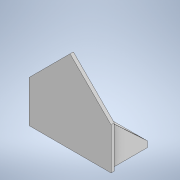
# Autodesk Inventor part: Halterung_ID6
Saved by Autodesk Inventor 2022.2 (Build 262287010, 287A)
## iProperties
Created: 2024-02-12
Part Number: Halterung_ID6
Material: Generisch
Document SubType Name: Modeling
Designer: ppovolni
Density: 1 g/cm^3
Appearance: Vorgabe
Author: ppovolni
Autodesk Inventor part; units mm, degrees
ref_plane "YZ Plane" through (0, 0, 0) normal (1, 0, 0) x (0, 1, 0)
ref_plane "XZ Plane" through (0, 0, 0) normal (0, 1, 0) x (-1, 0, 0)
ref_plane "XY Plane" through (0, 0, 0) normal (0, 0, 1) x (1, 0, 0)
sketch "Skizze1" plane through (0, 0, 0) normal (0, 0, 1) x (1, 0, 0)
  line L0 (0, 113.1371) -> (56.5685, 56.5685)
  line L1 (56.5685, 56.5685) -> (0, 0) construction
  line L2 (0, 0) -> (-56.5685, 56.5685) construction
  line L3 (-56.5685, 56.5685) -> (0, 113.1371)
  line L4 (0, 0) -> (-109.9706, 0) construction
  line L5 (-56.5685, 56.5685) -> (-56.5685, 0)
  line L6 (56.5685, 56.5685) -> (56.5685, 0)
  line L7 (-56.5685, 0) -> (56.5685, 0)
  dimension "d0" = 45
  dimension "d1" = 80
  constraints: 16 end point, 3 perpendicular, 2 horizontal, 2 parallel, 1 coincident, 1 point on line, 1 vertical
  measures "d0" angle of L4 L2
  measures "d1" distance of L0.end L1.end
extrude "Extrusion1" add sketch "Skizze1" along normal blind 5
sketch "Skizze2" plane through (0, 0, 0) normal (0, 0, -1) x (-1, 0, 0)
  line L0 (-56.5685, 0) -> (56.5685, 0)
  line L1 (56.5685, 0) -> (56.5685, 5)
  line L2 (56.5685, 5) -> (-56.5685, 5)
  line L3 (-56.5685, 5) -> (-56.5685, 0)
  line L4 (56.5685, 0) -> (-56.5685, 0) construction
  line L5 (56.5685, 56.5685) -> (56.5685, 0) construction
  line L6 (0, 113.1371) -> (56.5685, 56.5685) construction
  line L7 (-56.5685, 56.5685) -> (0, 113.1371) construction
  line L8 (-56.5685, 0) -> (-56.5685, 56.5685) construction
  point P0 (0, 0)
  dimension "d4" = 5
  constraints: 8 end point, 2 parallel, 1 collinear, 1 horizontal, 1 perpendicular
  measures "d4" distance between parallel lines of L0 L2
extrude "Extrusion2" add sketch "Skizze2" along normal blind 55
sketch "Skizze3" plane through (56.5685, 0, 5) normal (1, 0, 0) x (0, 0, -1)
  line L0 (5, 5) -> (5, 56.5685) construction
  line L1 (5, 5) -> (60, 5) construction
  line L2 (5, 56.5685) -> (60, 5)
  line L3 (60, 5) -> (5, 5)
  line L4 (5, 5) -> (5, 56.5685)
  point P0 (5, 0)
  constraints: 6 end point, 1 horizontal
extrude "Extrusion3" add sketch "Skizze3" against normal blind 5
sketch "Skizze4" plane through (-56.5685, 0, 5) normal (-1, 0, 0) x (0, 0, 1)
  line L0 (-5, 5) -> (-60, 5) projected
  line L1 (-5, 56.5685) -> (-5, 5) projected
  line L2 (-5, 56.5685) -> (-60, 5) projected
  point P0 (-5, 0)
extrude "Extrusion4" add sketch "Skizze4" against normal blind 5
sketch "Skizze5" plane through (51.5685, 5, 0) normal (0, 1, 0) x (1, 0, 0)
  line L0 (-15, 35) -> (-88.1371, 35) construction
  line L1 (-15, 38.1623) -> (-88.1371, 38.1623)
  line L2 (-88.1371, 31.8377) -> (-15, 31.8377)
  arc A0 (-15, 31.8377) -> (-15, 38.1623) centre (-15, 35) ccw
  arc A1 (-88.1371, 38.1623) -> (-88.1371, 31.8377) centre (-88.1371, 35) ccw
  line L3 (-103.1371, 55) -> (-103.1371, 0) construction
  line L4 (0, 0) -> (-103.1371, 0) construction
  line L5 (0, 0) -> (0, 55) construction
  line L6 (-103.1371, 55) -> (0, 55) construction
  point P0 (-51.5685, 0)
  point P1 (-51.5685, 35)
  dimension "d11" = 20
  dimension "d12" = 15
  dimension "d13" = 15
  constraints: 8 end point, 4 point on circle, 4 tangent, 2 centre point, 1 horizontal, 1 midpoint, 1 parallel
  measures "d11" distance between parallel lines of L6 L0
  measures "d12" distance from line of L5 L0.start
  measures "d13" distance from line of L0.end L3
extrude "Extrusion5" cut sketch "Skizze5" against normal through all
sketch "Skizze6" plane through (0, 0, 5) normal (0, 0, 1) x (1, 0, 0)
  line L0 (-56.5685, 0) -> (56.5685, 0) projected
  line L1 (56.5685, 0) -> (56.5685, 56.5685) projected
  line L2 (56.5685, 56.5685) -> (0, 113.1371) projected
  line L3 (0, 113.1371) -> (-56.5685, 56.5685) projected
  line L4 (-56.5685, 56.5685) -> (-56.5685, 0) projected
  line L5 (-61.5685, 58.6396) -> (0, 120.2082)
  line L6 (0, 120.2082) -> (61.5685, 58.6396)
  line L7 (61.5685, 58.6396) -> (61.5685, -4)
  line L8 (-61.5685, 58.6396) -> (-61.5685, -4)
  line L9 (-61.5685, -4) -> (61.5685, -4)
  line L10 (56.5685, 56.5685) -> (0, 113.1371) projected
  line L11 (-56.5685, 0) -> (56.5685, 0) projected
  point P0 (0, 0)
  dimension "d16" = 5
  dimension "d17" = 5
  dimension "d18" = 5
  dimension "d19" = 5
  dimension "d20" = 4
  constraints: 10 end point, 5 parallel, 1 perpendicular
  measures "d16" distance between parallel lines of L2 L6
  measures "d17" distance between parallel lines of L1 L7
  measures "d18" distance between parallel lines of L3 L5
  measures "d19" distance between parallel lines of L8 L4
  measures "d20" distance between parallel lines of L9 L0
extrude "Extrusion6" add sketch "Skizze6" against normal up to surface (5 mm away)
sketch "Skizze7" plane through (-56.5685, 0, 0) normal (0, -1, 0) x (1, 0, 0)
  line L0 (113.1371, 0) -> (0, 0) projected
  line L1 (0, 0) -> (0, -55) projected
  line L2 (113.1371, -55) -> (0, -55) projected
  line L3 (113.1371, -55) -> (113.1371, 0) projected
  line L4 (20, -31.8377) -> (93.1371, -31.8377) projected
  arc A0 (93.1371, -38.1623) -> (93.1371, -31.8377) centre (93.1371, -35) ccw projected
  line L5 (93.1371, -38.1623) -> (20, -38.1623) projected
  arc A1 (20, -31.8377) -> (20, -38.1623) centre (20, -35) ccw projected
  point P0 (56.5685, 0)
extrude "Extrusion7" add sketch "Skizze7" along normal blind 3.4
sketch "Skizze8" plane through (0, 0, -55) normal (0, 0, -1) x (-1, 0, 0)
  line L0 (56.5685, -3.4) -> (56.5685, 56.5685) construction
  line L1 (56.5685, -3.4) -> (-56.5685, -3.4) construction
  line L2 (-56.5685, -3.4) -> (-56.5685, 56.5685) construction
  line L3 (-56.5685, 56.5685) -> (-51.5685, 56.5685) construction
  line L4 (-51.5685, 56.5685) -> (-51.5685, 5) construction
  line L5 (-51.5685, 5) -> (51.5685, 5) construction
  line L6 (51.5685, 5) -> (51.5685, 56.5685) construction
  line L7 (51.5685, 56.5685) -> (56.5685, 56.5685) construction
  line L8 (0, 120.2082) -> (-61.5685, 58.6396) construction
  line L9 (-61.5685, 58.6396) -> (-61.5685, -4) construction
  line L10 (-61.5685, -4) -> (61.5685, -4) construction
  line L11 (61.5685, -4) -> (61.5685, 58.6396) construction
  line L12 (61.5685, 58.6396) -> (0, 120.2082) construction
  line L13 (96.047, 0) -> (96.047, 100) construction
  point P0 (0, 0)
  dimension "d25" = 96.047
  constraints: 2 end point, 1 vertical
  measures "d25" distance from line of L13 point (0, 0)
